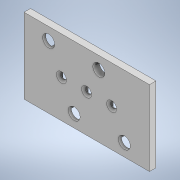
# Autodesk Inventor part: 1.27mmPitchProtoboard_nozzlePlate
Saved by Autodesk Inventor 2021 (Build 250183000, 183)
## iProperties
Created: 2022-02-04
Part Number: 1.27mmPitchProtoboard_nozzlePlate
Material: Generic
Document SubType Name: Modeling
Designer: Unit-005
Density: 1 g/cm^3
Appearance: Default
Author: Unit-005
## iProperties of the stored document _3DPrint.ipt
Created: 2022-02-04
Part Number: _3DPrint
Material: Generic
Document SubType Name: Modeling
Designer: Unit-005
Density: 1 g/cm^3
Appearance: Default
Author: Unit-005
Autodesk Inventor part; units mm, degrees
ref_plane "YZ Plane" through (0, 0, 0) normal (1, 0, 0) x (0, 1, 0)
ref_plane "XZ Plane" through (0, 0, 0) normal (0, 1, 0) x (-1, 0, 0)
ref_plane "XY Plane" through (0, 0, 0) normal (0, 0, 1) x (1, 0, 0)
sketch "Sketch1" plane through (0, 0, 0) normal (0, 0, 1) x (1, 0, 0)
  line L0 (-3.175, 1.905) -> (3.175, 1.905)
  line L1 (3.175, 1.905) -> (3.175, -1.905)
  line L2 (3.175, -1.905) -> (-3.175, -1.905)
  line L3 (-3.175, -1.905) -> (-3.175, 1.905)
  line L4 (-3.175, 1.905) -> (3.175, -1.905) construction
  line L5 (3.175, 1.905) -> (-3.175, -1.905) construction
  point P0 (0, 0)
  dimension "d0" = 6.35
  dimension "d1" = 3.81
  constraints: 12 end point, 2 midpoint, 2 parallel, 1 horizontal, 1 perpendicular
  measures "d0" distance of L1.end L2.end
  measures "d1" distance between parallel lines of L2 L0
sketch "Sketch1 outline for Extrusion1" plane through (0, 0, 0) normal (0, 0, 1) x (1, 0, 0)
  line L0 (-3.175, 1.905) -> (-3.175, -1.905)
  line L1 (3.175, 1.905) -> (-3.175, 1.905)
  line L2 (3.175, -1.905) -> (3.175, 1.905)
  line L3 (-3.175, -1.905) -> (3.175, -1.905)
extrude "Extrusion1" add sketch "Sketch1 outline for Extrusion1" along normal blind 0.15
sketch "Sketch2" plane through (0, 0, 0) normal (0, 0, -1) x (-1, 0, 0)
  line L0 (-3.0353, 1.7653) -> (3.0353, 1.7653)
  line L1 (3.0353, 1.7653) -> (3.0353, -1.7653)
  line L2 (3.0353, -1.7653) -> (-3.0353, -1.7653)
  line L3 (-3.0353, -1.7653) -> (-3.0353, 1.7653)
  line L4 (-3.0353, 1.7653) -> (3.0353, -1.7653) construction
  line L5 (3.0353, 1.7653) -> (-3.0353, -1.7653) construction
  line L6 (3.175, -1.905) -> (-3.175, -1.905) projected
  line L7 (3.175, 1.905) -> (3.175, -1.905) projected
  line L8 (-3.175, 1.905) -> (3.175, 1.905) projected
  line L9 (-3.175, -1.905) -> (-3.175, 1.905) projected
  line L10 (4.445, 0) -> (-4.445, 0) projected
  line L11 (0, -2.667) -> (0, 2.667) projected
  line L12 (2.4511, -1.7653) -> (2.1971, -1.7653)
  line L13 (2.1971, -1.7653) -> (2.1971, 1.7653)
  line L14 (2.1971, 1.7653) -> (2.4511, 1.7653)
  line L15 (2.4511, 1.7653) -> (2.4511, -1.7653)
  line L16 (2.4511, -1.7653) -> (2.1971, 1.7653) construction
  line L17 (2.1971, -1.7653) -> (2.4511, 1.7653) construction
  line L18 (1.3971, -1.7653) -> (1.3971, 1.7653)
  line L19 (1.6511, 1.7653) -> (1.6511, -1.7653)
  line L20 (-2.4511, -1.7653) -> (-2.1971, -1.7653)
  line L21 (-2.1971, -1.7653) -> (-2.1971, 1.7653)
  line L22 (-2.1971, 1.7653) -> (-2.4511, 1.7653)
  line L23 (-2.4511, 1.7653) -> (-2.4511, -1.7653)
  line L24 (-2.4511, -1.7653) -> (-2.1971, 1.7653) construction
  line L25 (-2.1971, -1.7653) -> (-2.4511, 1.7653) construction
  line L26 (-1.3971, -1.7653) -> (-1.3971, 1.7653)
  line L27 (-1.6511, 1.7653) -> (-1.6511, -1.7653)
  line L28 (0.2667, 1.7653) -> (0.5207, 1.7653)
  line L29 (-0.2793, 1.7653) -> (-0.2793, -1.7653)
  line L30 (0.2667, -1.7653) -> (0.2667, 1.7653)
  line L31 (0.5207, -1.7653) -> (0.2667, -1.7653)
  line L32 (0.5207, -1.7653) -> (0.2667, 1.7653) construction
  line L33 (0.2667, -1.7653) -> (0.5207, 1.7653) construction
  line L34 (0.5207, 1.7653) -> (0.5207, -1.7653)
  line L35 (-0.5333, -1.7653) -> (-0.5333, 1.7653)
  point P0 (0, 0)
  point P1 (2.3241, 0)
  point P2 (-2.3241, 0)
  point P3 (0.3937, 0)
  point P4 (2.4511, 0)
  point P5 (2.1971, 0)
  point P6 (1.6511, 0)
  point P7 (1.3971, 0)
  point P8 (0.5207, 0)
  point P9 (0.2667, 0)
  point P10 (-0.5333, 0)
  point P11 (-0.2793, 0)
  point P12 (-1.6511, 0)
  point P13 (-1.3971, 0)
  point P14 (-2.4511, 0)
  point P15 (-2.1971, 0)
  dimension "d4" = 6.0706
  dimension "d5" = 3.5306
  dimension "d8" = 0.254
  dimension "d9" = 0.8509
  dimension "d12" = 0.8
  dimension "d45" = 1.9304
  constraints: 60 end point, 9 symmetric about line, 8 midpoint, 4 horizontal, 4 parallel, 2 perpendicular, 2 point on line, 23 other
  measures "d4" distance of L1.end L2.end
  measures "d5" distance of L0.end L1.end
  measures "d8" distance of L13.end L14.end
  measures "d9" distance from line of L7 point (2.324, 0)
  measures "d12" distance of L12.end L18.start
  measures "d45" distance of L13.end L28.start
sketch "Sketch2 outline for Extrusion2" plane through (0, 0, 0) normal (0, 0, -1) x (-1, 0, 0)
  line L0 (3.175, -1.905) -> (3.175, 1.905)
  line L1 (-3.175, -1.905) -> (3.175, -1.905)
  line L2 (3.175, 1.905) -> (-3.175, 1.905)
  line L3 (-3.175, 1.905) -> (-3.175, -1.905)
  line L4 (-3.0353, 1.7653) -> (3.0353, 1.7653)
  line L5 (-3.0353, -1.7653) -> (-3.0353, 1.7653)
  line L6 (3.0353, -1.7653) -> (-3.0353, -1.7653)
  line L7 (3.0353, 1.7653) -> (3.0353, -1.7653)
extrude "Extrusion2" add sketch "Sketch2 outline for Extrusion2" along normal blind 0.18
sketch "Sketch3" plane through (0, 0, 0.15) normal (0, 0, 1) x (1, 0, 0)
  line L0 (-3.175, -1.905) -> (3.175, -1.905) projected
  line L1 (3.175, -1.905) -> (3.175, 1.905) projected
  line L2 (3.175, 1.905) -> (-3.175, 1.905) projected
  line L3 (-3.175, 1.905) -> (-3.175, -1.905) projected
  line L4 (-4.445, 0) -> (4.445, 0) projected
  line L5 (0, 2.667) -> (0, -2.667) projected
  circle A0 centre (-1.28, 0) radius 0.1524
  circle A1 centre (-0.01, 0) radius 0.1524
  circle A2 centre (1.26, 0) radius 0.1524
  point P0 (0, 0)
  dimension "d17" = 0.3048
  dimension "d18" = 1.895
  dimension "d21" = 1.27
  constraints: 3 centre point, 1 horizontal, 1 point on line, 4 other
  measures "d17" diameter of A0
  measures "d18" distance from line of L3 A0.centre
  measures "d21" distance of A0.centre A1.centre
sketch "Sketch3 outline for Extrusion3" plane through (0, 0, 0.15) normal (0, 0, 1) x (1, 0, 0)
  circle A0 centre (1.26, 0) radius 0.1524
  circle A1 centre (-0.01, 0) radius 0.1524
  circle A2 centre (-1.28, 0) radius 0.1524
extrude "Extrusion3" cut sketch "Sketch3 outline for Extrusion3" against normal through all
chamfer "Chamfer1" distance 0.1016 angle 45 3 edges at (-0.1624, 0, 0.15) (-1.4324, 0, 0.15) (1.1076, 0, 0.15)
sketch "Sketch4" plane through (2.4511, -1.7653, 0) normal (1, 0, 0) x (0, 0, -1)
  line L0 (0.18, 3.5306) -> (0.18, 1.7653) projected
  line L1 (0, 1.7653) -> (0, 3.5306) projected
  line L2 (0, 3.5306) -> (0.18, 3.5306) projected
  line L3 (0, 0) -> (0.18, 0) projected
  line L4 (0, 1.7653) -> (0.18, 1.7653)
  line L5 (0.18, 0) -> (0.18, 3.5306) projected
  line L6 (0.13, 1.7653) -> (0.18, 1.7153)
  line L7 (0.13, 1.7653) -> (0.18, 1.8153)
  line L8 (0.18, 1.8153) -> (0.18, 1.7153)
  dimension "d31" = 0.05
  dimension "d32" = 0.05
  constraints: 8 end point, 2 point on line, 1 collinear, 1 midpoint, 1 symmetric about line
  measures "d31" distance from line of L0 L6.start
  measures "d32" distance from line of L4 L6.end
extrude "Extrusion4" [suppressed]
sketch "Sketch5" plane through (0, 0, 0.15) normal (0, 0, 1) x (1, 0, 0)
  circle A0 centre (-1.28, 0) radius 0.254 projected
  line L0 (-3.175, -1.905) -> (3.175, -1.905) projected
  line L1 (3.175, -1.905) -> (3.175, 1.905) projected
  line L2 (3.175, 1.905) -> (-3.175, 1.905) projected
  line L3 (-3.175, 1.905) -> (-3.175, -1.905) projected
  circle A1 centre (-0.01, 0) radius 0.254 projected
  circle A2 centre (1.26, 0) radius 0.254 projected
  line L4 (-4.445, 0) -> (4.445, 0) projected
  line L5 (0, -2.667) -> (0, 2.667) projected
  circle A3 centre (1.905, -1.27) radius 0.3
  point P0 (0, 0)
  dimension "d35" = 0.6
  dimension "d36" = 1.27
  dimension "d37" = 1.27
  constraints: 1 centre point
  measures "d35" diameter of A3
  measures "d36" distance from line of L1 A3.centre
  measures "d37" distance from line of L4 A3.centre
sketch "Sketch5 outline for Extrusion5" plane through (0, 0, 0.15) normal (0, 0, 1) x (1, 0, 0)
  circle A0 centre (1.905, -1.27) radius 0.3
extrude "Extrusion5" cut sketch "Sketch5 outline for Extrusion5" against normal through all
pattern_linear "Rectangular Pattern1" count 2 spacing 2.54 along (-1, 0, 0) of "Extrusion5"
sketch "Sketch6" plane through (0, 0, 0) normal (0, 0, -1) x (-1, 0, 0)
  circle A0 centre (0.635, -1.27) radius 0.3
  circle A1 centre (-1.905, -1.27) radius 0.3
  circle A2 centre (-1.26, 0) radius 0.1524
  circle A3 centre (0.01, 0) radius 0.1524
  circle A4 centre (1.28, 0) radius 0.1524
  line L0 (-3.0353, 1.7653) -> (-3.0353, -1.7653)
  line L1 (-3.0353, -1.7653) -> (3.0353, -1.7653)
  line L2 (3.0353, -1.7653) -> (3.0353, 1.7653)
  line L3 (3.0353, 1.7653) -> (-3.0353, 1.7653)
  line L4 (4.445, 0) -> (-4.445, 0)
  line L5 (0, -2.667) -> (0, 2.667)
  line L6 (3.175, 1.905) -> (-3.175, 1.905)
  line L7 (-3.175, 1.905) -> (-3.175, -1.905)
  line L8 (-3.175, -1.905) -> (3.175, -1.905)
  line L9 (3.175, -1.905) -> (3.175, 1.905)
  line L10 (-3.0353, 1.7653) -> (3.0353, 1.7653)
  line L11 (3.0353, 1.7653) -> (3.0353, -1.7653)
  line L12 (3.0353, -1.7653) -> (-3.0353, -1.7653)
  line L13 (-3.0353, -1.7653) -> (-3.0353, 1.7653)
  line L14 (-1.514, 1.27) -> (-1.905, 1.27)
  line L15 (-1.905, 1.27) -> (-1.905, -1.27)
  line L16 (-1.905, -1.27) -> (-1.514, -1.27)
  line L17 (-1.514, -1.27) -> (-1.514, 1.27)
  line L18 (-1.514, 1.27) -> (-1.905, -1.27) construction
  line L19 (-1.905, 1.27) -> (-1.514, -1.27) construction
  circle A5 centre (-1.905, 1.27) radius 0.3
  line L20 (-1.26, 0.717103) -> (-1.26, -0.717103)
  line L21 (-1.006, 1.27) -> (-0.615, 1.27)
  line L22 (-0.615, 1.27) -> (-0.615, -1.27)
  line L23 (-0.615, -1.27) -> (-1.006, -1.27)
  line L24 (-1.006, -1.27) -> (-1.006, 1.27)
  line L25 (-1.006, 1.27) -> (-0.615, -1.27) construction
  line L26 (-0.615, 1.27) -> (-1.006, -1.27) construction
  circle A6 centre (-0.615, -1.27) radius 0.3048
  circle A7 centre (-0.615, 1.27) radius 0.3048
  point P0 (0, 0)
  point P1 (-1.7095, 0)
  point P2 (-1.7095, 1.27)
  point P3 (-0.8105, 0)
  point P4 (-0.8105, 1.27)
  point P5 (-0.935, -1.27)
  point P6 (-0.615, -0.970667)
  point P7 (-1.905, -0.97)
  point P8 (-1.605, -1.27)
  point P9 (-0.615, 0.9652)
  point P10 (-0.9198, 1.27)
  point P11 (-0.9198, -1.27)
  point P12 (-0.615, -0.9652)
  point P13 (-1.605, 1.27)
  point P14 (-1.905, 0.97)
  dimension "d52" = 0.254
  dimension "d54" = 1.43421
  dimension "d63" = 0.6096
  constraints: 26 end point, 9 symmetric about line, 6 midpoint, 2 centre point, 2 coincident, 2 parallel, 1 horizontal, 1 perpendicular, 1 point on line, 1 vertical, 1 other
  measures "d52" distance from line of L17 A2.centre
  measures "d54" distance of L20.start L20.end
  measures "d63" diameter of A6
sketch "Sketch6 outline for Extrusion6" plane through (0, 0, 0) normal (0, 0, -1) x (-1, 0, 0)
  arc A0 (-0.615, 0.9652) -> (-0.9198, 1.27) centre (-0.615, 1.27) cw
  line L0 (-0.615, -0.9652) -> (-0.615, 0.9652)
  arc A1 (-0.9198, -1.27) -> (-0.615, -0.9652) centre (-0.615, -1.27) cw
  line L1 (-1.006, -1.27) -> (-0.9198, -1.27)
  line L2 (-1.006, 1.27) -> (-1.006, -1.27)
  line L3 (-0.9198, 1.27) -> (-1.006, 1.27)
  arc A2 (-1.605, 1.27) -> (-1.905, 0.97) centre (-1.905, 1.27) cw
  line L4 (-1.514, 1.27) -> (-1.605, 1.27)
  line L5 (-1.514, -1.27) -> (-1.514, 1.27)
  line L6 (-1.605, -1.27) -> (-1.514, -1.27)
  arc A3 (-1.905, -0.97) -> (-1.605, -1.27) centre (-1.905, -1.27) cw
  line L7 (-1.905, 0.97) -> (-1.905, -0.97)
extrude "Extrusion6" add sketch "Sketch6 outline for Extrusion6" along normal blind 0.18
pattern_linear "Rectangular Pattern2" count 3 spacing 1.27 along (-1, 0, 0) of "Extrusion6"
chamfer "Chamfer2" distance 0.1778 angle 45 4 edges at (0, -1.7653, 0) (-3.0353, 0, 0) (0, 1.7653, 0) (3.0353, 0, 0)
sketch "Sketch7" plane through (0, 0, 0) normal (0, 0, -1) x (-1, 0, 0)
  line L0 (1.6202, 1.27) -> (1.534, 1.27)
  line L1 (1.534, 1.27) -> (1.534, -1.27)
  line L2 (1.534, -1.27) -> (1.6202, -1.27)
  arc A0 (1.925, -0.9652) -> (1.6202, -1.27) centre (1.925, -1.27) ccw
  line L3 (1.925, -0.9652) -> (1.925, 0.9652)
  arc A1 (1.6202, 1.27) -> (1.925, 0.9652) centre (1.925, 1.27) ccw
  arc A2 (-0.9198, 1.27) -> (-0.635, 0.965857) centre (-0.615, 1.27) ccw
  line L4 (-0.9198, 1.27) -> (-1.006, 1.27)
  line L5 (-1.006, 1.27) -> (-1.006, -1.27)
  line L6 (-1.006, -1.27) -> (-0.9198, -1.27)
  arc A3 (-0.635, -0.965857) -> (-0.9198, -1.27) centre (-0.615, -1.27) ccw
  line L7 (-0.635, -0.965857) -> (-0.635, -0.97)
  arc A4 (-0.335, -1.27) -> (-0.635, -0.97) centre (-0.635, -1.27) ccw
  line L8 (-0.335, -1.27) -> (-0.244, -1.27)
  line L9 (-0.244, -1.27) -> (-0.244, 1.27)
  line L10 (-0.244, 1.27) -> (-0.335, 1.27)
  line L11 (-0.635, 0.97) -> (-0.635, 0.965857)
  line L12 (1.026, -1.27) -> (0.935, -1.27)
  arc A5 (0.335, -1.27) -> (0.935, -1.27) centre (0.635, -1.27) ccw
  line L13 (0.335, -1.27) -> (0.264, -1.27)
  line L14 (0.264, -1.27) -> (0.264, 1.27)
  line L15 (0.264, 1.27) -> (0.3502, 1.27)
  arc A6 (0.3502, 1.27) -> (0.635, 0.965857) centre (0.655, 1.27) ccw
  line L16 (0.635, 0.965857) -> (0.635, 0.97)
  line L17 (0.935, 1.27) -> (1.026, 1.27)
  line L18 (1.026, 1.27) -> (1.026, -1.27)
  arc A7 (1.6202, 1.27) -> (1.925, 0.9652) centre (1.925, 1.27) ccw
  line L19 (1.925, 0.9652) -> (1.925, -0.9652)
  arc A8 (1.925, -0.9652) -> (1.6202, -1.27) centre (1.925, -1.27) ccw
  line L20 (1.6202, -1.27) -> (1.534, -1.27)
  line L21 (1.534, -1.27) -> (1.534, 1.27)
  line L22 (1.534, 1.27) -> (1.6202, 1.27)
  line L23 (-1.514, -1.27) -> (-1.605, -1.27)
  arc A9 (-1.905, -0.97) -> (-1.605, -1.27) centre (-1.905, -1.27) ccw
  line L24 (-1.905, -0.97) -> (-1.905, 0.97)
  line L25 (-1.605, 1.27) -> (-1.514, 1.27)
  line L26 (-1.514, 1.27) -> (-1.514, -1.27)
  line L27 (-0.635, 0.965857) -> (-0.635, 0.97)
  line L28 (-0.335, 1.27) -> (-0.244, 1.27)
  line L29 (-0.244, 1.27) -> (-0.244, -1.27)
  line L30 (-0.244, -1.27) -> (-0.335, -1.27)
  arc A10 (-0.335, -1.27) -> (-0.635, -0.97) centre (-0.635, -1.27) ccw
  line L31 (-0.635, -0.97) -> (-0.635, -0.965857)
  arc A11 (-0.635, -0.965857) -> (-0.9198, -1.27) centre (-0.615, -1.27) ccw
  line L32 (-0.9198, -1.27) -> (-1.006, -1.27)
  line L33 (-1.006, -1.27) -> (-1.006, 1.27)
  line L34 (-1.006, 1.27) -> (-0.9198, 1.27)
  arc A12 (-0.9198, 1.27) -> (-0.635, 0.965857) centre (-0.615, 1.27) ccw
  circle A13 centre (-1.26, 0) radius 0.1524
  circle A14 centre (0.01, 0) radius 0.1524
  circle A15 centre (1.28, 0) radius 0.1524
  line L35 (-2.8575, -1.5875) -> (-2.8575, 1.5875)
  line L36 (2.8575, -1.5875) -> (-2.8575, -1.5875)
  line L37 (2.8575, 1.5875) -> (2.8575, -1.5875)
  line L38 (-2.8575, 1.5875) -> (2.8575, 1.5875)
  line L39 (3.175, 1.905) -> (-3.175, 1.905)
  line L40 (-3.175, 1.905) -> (-3.175, -1.905)
  line L41 (-3.175, -1.905) -> (3.175, -1.905)
  line L42 (3.175, -1.905) -> (3.175, 1.905)
  line L43 (-3.0353, 1.7653) -> (3.0353, 1.7653)
  line L44 (3.0353, 1.7653) -> (3.0353, -1.7653)
  line L45 (3.0353, -1.7653) -> (-3.0353, -1.7653)
  line L46 (-3.0353, -1.7653) -> (-3.0353, 1.7653)
  arc A16 (1.6202, 1.27) -> (1.925, 0.9652) centre (1.925, 1.27) ccw
  circle A17 centre (1.925, 1.27) radius 0.3048
  circle A18 centre (-0.615, 1.27) radius 0.3048
  arc A19 (0.3502, 1.27) -> (0.635, 0.965857) centre (0.655, 1.27) ccw
  circle A20 centre (0.635, 1.27) radius 0.2848
  arc A21 (-0.635, 0.97) -> (-0.335, 1.27) centre (-0.635, 1.27) ccw
  line L47 (0.635, -0.97) -> (0.635, -0.965857)
  arc A22 (0.635, -0.965857) -> (0.572424, -0.976599) centre (0.655, -1.27) ccw
  arc A23 (0.635, -0.97) -> (0.572424, -0.976599) centre (0.635, -1.27) ccw
  arc A24 (0.635, 0.97) -> (0.935, 1.27) centre (0.635, 1.27) ccw
  arc A25 (-1.905, 0.97) -> (-1.605, 1.27) centre (-1.905, 1.27) ccw
  arc A26 (-0.635, 0.97) -> (-0.335, 1.27) centre (-0.635, 1.27) ccw
  point P0 (0, 0)
  point P1 (-0.9198, 1.27)
  dimension "d66" = 2.54
  constraints: 2 horizontal, 1 coincident, 1 horizontal alignment, 11 other
  measures "d66" distance of point (1.925, 1.27) point (-0.615, 1.27)
sketch "Sketch7 outline for Extrusion7" plane through (0, 0, 0) normal (0, 0, -1) x (-1, 0, 0)
  circle A0 centre (-0.615, 1.27) radius 0.3048
  circle A1 centre (1.925, 1.27) radius 0.3048
extrude "Extrusion7" cut sketch "Sketch7 outline for Extrusion7" against normal through all both and the other way through all
body "Solid1"
